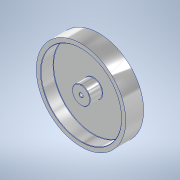
# Autodesk Inventor part: felge
Saved by Autodesk Inventor 2022 (Build 260153000, 153)
## iProperties
Created: 2022-11-16
Part Number: felge
Material: Aluminium 6061
Document SubType Name: Modeling
Designer: Friedrich Walmrath
Density: 2.7 g/cm^3
Appearance: Aluminium - flach
Mass: 24.3488 g
Surface Area: 67.2741 cm^2
Volume: 9.01806 cm^3
Author: Friedrich Walmrath
Autodesk Inventor part; units mm, degrees
ref_plane "YZ Plane" through (0, 0, 0) normal (1, 0, 0) x (0, 1, 0)
ref_plane "XZ Plane" through (0, 0, 0) normal (0, 1, 0) x (-1, 0, 0)
ref_plane "XY Plane" through (0, 0, 0) normal (0, 0, 1) x (1, 0, 0)
sketch "Skizze1" plane through (0, 0, 0) normal (0, 0, 1) x (1, 0, 0)
  circle A0 centre (0, 0) radius 30
  dimension "d0" = 60
  constraints: 1 centre point, 1 coincident
  measures "d0" diameter of A0
extrude "Extrusion1" add sketch "Skizze1" along normal blind 10
sketch "Skizze2" plane through (0, 0, 10) normal (0, 0, 1) x (1, 0, 0)
  circle A0 centre (0, 0) radius 30 projected
  circle A1 centre (0, 0) radius 22.5
  circle A2 centre (0, 0) radius 5
  dimension "d3" = 7.5
  dimension "d4" = 10
  constraints: 2 centre point, 1 coincident
  measures "d3" radial gap between concentric circles of A0 A1
  measures "d4" diameter of A2
extrude "Extrusion2" cut sketch "Skizze2" against normal blind 7 contours A1
sketch "Skizze3" plane through (0, 0, 10) normal (0, 0, 1) x (1, 0, 0)
  circle A0 centre (0, 0) radius 1
  dimension "d7" = 2
  constraints: 1 centre point, 1 coincident
  measures "d7" diameter of A0
extrude "Extrusion3" cut sketch "Skizze3" along normal through all both and the other way through all
fillet "Rundung1" radius 0.2 2 edges at (-22.5, 0, 3) (-5, 0, 3)
chamfer "Fase1" distance 0.2 angle 45 6 edges at (-30, 0, 0) (-30, 0, 10) (-22.5, 0, 10) (-5, 0, 10) (-1, 0, 10) (-1, 0, 0)
sketch "Skizze4" plane through (0, 0, 10) normal (0, 0, 1) x (1, 0, 0)
  circle A0 centre (0, 0) radius 25
  circle A1 centre (0, 0) radius 40
  dimension "d14" = 50
  dimension "d15" = 15
  constraints: 2 centre point, 1 coincident
  measures "d14" diameter of A0
  measures "d15" radial gap between concentric circles of A0 A1
extrude "Extrusion4" cut sketch "Skizze4" along normal through all both and the other way through all
sketch "Skizze5" plane through (0, 0, 10) normal (0, 0, 1) x (1, 0, 0)
  circle A0 centre (0, 0) radius 1.2 projected
  circle A1 centre (0, 0) radius 27.5
  circle A2 centre (0, 0) radius 30
  dimension "d18" = 55
  dimension "d19" = 60
  constraints: 2 centre point, 2 coincident
  measures "d18" diameter of A1
  measures "d19" diameter of A2
